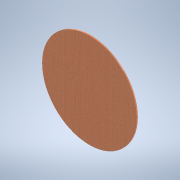
# Autodesk Inventor part: Drehteller
Saved by Autodesk Inventor 2021 (Build 250183000, 183)
## iProperties
Created: 2022-06-25
Part Number: Drehteller
Material: Holz (Eiche)
Document SubType Name: Modeling
Designer: adria
Mass: 477.522 g
Surface Area: 2576.11 cm^2
Volume: 628.319 cm^3
Density: 0.76 g/cm^3
Appearance: Weißeiche - natur - mittlerer Glanz
Author: adria
Autodesk Inventor part; units mm, degrees
ref_plane "YZ Plane" through (0, 0, 0) normal (1, 0, 0) x (0, 1, 0)
ref_plane "XZ Plane" through (0, 0, 0) normal (0, 1, 0) x (-1, 0, 0)
ref_plane "XY Plane" through (0, 0, 0) normal (0, 0, 1) x (1, 0, 0)
sketch "Skizze1" plane through (0, 0, 0) normal (0, 0, 1) x (1, 0, 0)
  circle A0 centre (0, 0) radius 200
  dimension "d0" = 400
  constraints: 1 centre point, 1 coincident
  measures "d0" diameter of A0
extrude "Extrusion1" add sketch "Skizze1" along normal blind 5
sketch "Skizze2" plane through (0, 0, 5) normal (0, 0, 1) x (1, 0, 0)
  circle A0 centre (0, 0) radius 200 projected
  line L0 (-280, 0) -> (280, 0) projected
  line L1 (0, -280) -> (0, 280) projected
  point P0 (0, 75)
  point P1 (-75, 0)
  point P2 (0, -75)
  point P3 (75, 0)
  dimension "d3" = 75
  dimension "d6" = 360
  constraints: 1 point on line, 5 other
  measures "d3" distance from line of L0 point (0, 75)
